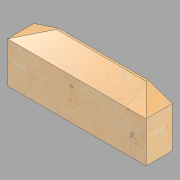
# Autodesk Inventor part: Straight_cap_7
Saved by Autodesk Inventor 2022.2 (Build 262287010, 287A)
## iProperties
Created: 2021-12-03
Part Number: Straight_cap_7
Material: Limestone
Document SubType Name: Modeling
Designer: awelt
Density: 2.6 g/cm^3
Appearance: Kasota Gray
Mass: 103022 g
Surface Area: 8511.98 cm^2
Volume: 39623.9 cm^3
Author: awelt
Autodesk Inventor part; units mm, degrees
ref_plane "YZ Plane" through (0, 0, 0) normal (1, 0, 0) x (0, 1, 0)
ref_plane "XZ Plane" through (0, 0, 0) normal (0, 1, 0) x (-1, 0, 0)
ref_plane "XY Plane" through (0, 0, 0) normal (0, 0, 1) x (1, 0, 0)
sketch "Sketch1" plane through (0, 0, 0) normal (0, 1, 0) x (-1, 0, 0)
  line L0 (431.8, -82.55) -> (-431.8, -82.55)
  line L1 (-431.8, -82.55) -> (-431.8, 82.55)
  line L2 (-431.8, 82.55) -> (431.8, 82.55)
  line L3 (431.8, 82.55) -> (431.8, -82.55)
  line L4 (431.8, -82.55) -> (-431.8, 82.55) construction
  line L5 (-431.8, -82.55) -> (431.8, 82.55) construction
  point P0 (0, 0)
  dimension "d0" = 863.6
  dimension "d1" = 165.1
  constraints: 12 end point, 2 midpoint, 2 parallel, 1 horizontal, 1 perpendicular
  measures "d0" distance of L1.end L2.end
  measures "d1" distance of L0.end L1.end
extrude "Extrusion1" add sketch "Sketch1" along normal blind 304.8
sketch "Sketch2" plane through (431.8, 0, 82.55) normal (1, 0, 0) x (0, 0, -1)
  line L0 (0, 304.8) -> (165.1, 304.8) projected
  line L1 (165.1, 0) -> (165.1, 304.8) projected
  line L2 (12.7, 304.8) -> (165.1, 254)
  line L3 (165.1, 254) -> (165.1, 304.8)
  line L4 (165.1, 304.8) -> (12.7, 304.8)
  point P0 (82.55, 0)
  dimension "d4" = 12.7
  dimension "d5" = 50.8
  constraints: 6 end point, 2 point on line, 1 collinear, 1 perpendicular
  measures "d4" distance of L2.start L0.start
  measures "d5" distance of L2.end L0.end
extrude "Extrusion2" cut sketch "Sketch2" against normal through all
sketch "Sketch3" plane through (-431.8, 0, 82.55) normal (0, 0, 1) x (1, 0, 0)
  line L0 (0, 304.8) -> (863.6, 304.8) projected
  line L1 (863.6, 0) -> (863.6, 304.8) projected
  line L2 (431.8, 304.8) -> (431.8, 0) construction
  line L3 (863.6, 0) -> (0, 0) construction
  line L4 (711.2, 304.8) -> (863.6, 254)
  line L5 (152.4, 304.8) -> (0, 254)
  line L6 (0, 0) -> (0, 304.8) projected
  line L7 (0, 254) -> (0, 304.8)
  line L8 (0, 304.8) -> (152.4, 304.8)
  dimension "d8" = 152.4
  dimension "d9" = 50.8
  constraints: 10 end point, 2 collinear, 2 point on line, 2 symmetric about line, 1 midpoint, 1 perpendicular
  measures "d8" distance of L4.start L0.end
  measures "d9" distance of L4.end L0.end
extrude "Extrusion3" cut sketch "Sketch3" against normal through all contours L0 L1 L4
extrude "Extrusion4" cut sketch "Sketch3" against normal through all contours L0 L5 L6
body "Solid1"
